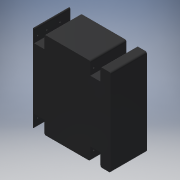
# Autodesk Inventor part: Part2
Saved by Autodesk Inventor 2016 (Build 200138000, 138)
## iProperties
Created: 2015-06-07
Part Number: Part2
Material: ABS Plastic
Document SubType Name: Sheet Metal
Designer: Jufo
Density: 1 g/cm^3
Sheet Metal Rule: Default
Appearance: Smooth - White
Author: Jufo
Autodesk Inventor part; units mm, degrees
ref_plane "YZ Plane" through (0, 0, 0) normal (1, 0, 0) x (0, 1, 0)
ref_plane "XZ Plane" through (0, 0, 0) normal (0, 1, 0) x (-1, 0, 0)
ref_plane "XY Plane" through (0, 0, 0) normal (0, 0, 1) x (1, 0, 0)
sketch "Sketch1" plane through (0, 0, 0) normal (0, 1, 0) x (-1, 0, 0)
  line L0 (65.7605, 110.8282) -> (65.7605, 85.8282)
  line L1 (65.7605, 85.8282) -> (45.7605, 85.8282)
  line L2 (45.7605, 85.8282) -> (45.7605, 110.8282)
  line L3 (45.7605, 110.8282) -> (-44.2395, 110.8282)
  line L4 (-44.2395, 110.8282) -> (-44.2395, 85.8282)
  line L5 (-44.2395, 85.8282) -> (-64.2395, 85.8282)
  line L6 (-64.2395, 85.8282) -> (-64.2395, 110.8282)
  line L7 (-64.2395, 110.8282) -> (-84.2395, 110.8282)
  line L8 (-84.2395, 110.8282) -> (-84.2395, -59.1718)
  line L9 (-84.2395, -59.1718) -> (-64.2395, -59.1718)
  line L10 (-64.2395, -59.1718) -> (-64.2395, -34.1718)
  line L11 (-64.2395, -34.1718) -> (-44.2395, -34.1718)
  line L12 (-44.2395, -34.1718) -> (-44.2395, -59.1718)
  line L13 (-44.2395, -59.1718) -> (45.7605, -59.1718)
  line L14 (45.7605, -59.1718) -> (45.7605, -34.1718)
  line L15 (45.7605, -34.1718) -> (65.7605, -34.1718)
  line L16 (65.7605, -34.1718) -> (65.7605, -59.1718)
  line L17 (65.7605, 110.8282) -> (67.7605, 110.8282)
  line L18 (67.7605, 110.8282) -> (67.7605, -59.1718)
  line L19 (67.7605, -59.1718) -> (65.7605, -59.1718)
  point P0 (0, 0)
  dimension "d0" = 2
  dimension "d1" = 20
  dimension "d2" = 20
  dimension "d3" = 170
  dimension "d4" = 170
  dimension "d6" = 25
  dimension "d9" = 25
  dimension "d10" = 25
  dimension "d11" = 25
  dimension "d12" = 20
  dimension "d13" = 90
  dimension "d14" = 20
  dimension "d15" = 2
  dimension "d16" = 90
  dimension "d17" = 20
  dimension "d113" = 25
  dimension "d114" = 25
  dimension "d115" = 25
  constraints: 40 end point, 14 parallel, 3 perpendicular, 2 collinear, 1 vertical
  measures "d0" distance of L0.start L17.end
  measures "d1" distance of L14.end L15.end
  measures "d2" distance of L0.end L1.end
  measures "d3" distance of L17.end L18.end
  measures "d4" distance of L7.end L8.end
  measures "d6" distance of L13.end L14.end
  measures "d9" distance of L5.end L6.end
  measures "d10" distance of L9.end L10.end
  measures "d11" distance of L11.end L12.end
  measures "d12" distance of L6.end L7.end
  measures "d13" distance of L2.end L3.end
  measures "d14" distance of L8.end L9.end
  measures "d15" distance of L18.end L16.end
  measures "d16" distance of L12.end L13.end
  measures "d17" distance of L10.end L11.end
  measures "d113" distance of L1.end L2.end
  measures "d114" distance of L3.end L4.end
  measures "d115" distance of L0.start L0.end
extrude "Extrusion1" add sketch "Sketch1" along normal blind 2
sketch "Sketch2" plane through (0, 2, 0) normal (0, 1, 0) x (1, 0, 0)
  line L0 (-65.7605, -110.8282) -> (-65.7605, -85.8282) projected
  line L1 (-65.7605, -85.8282) -> (-45.7605, -85.8282) projected
  line L2 (-45.7605, -85.8282) -> (-45.7605, -110.8282) projected
  line L3 (-45.7605, -110.8282) -> (44.2395, -110.8282) projected
  line L4 (44.2395, -110.8282) -> (44.2395, -85.8282) projected
  line L5 (44.2395, -85.8282) -> (64.2395, -85.8282) projected
  line L6 (64.2395, -85.8282) -> (64.2395, -110.8282) projected
  line L7 (64.2395, -110.8282) -> (84.2395, -110.8282) projected
  line L8 (84.2395, -110.8282) -> (84.2395, 59.1718) projected
  line L9 (84.2395, 59.1718) -> (64.2395, 59.1718) projected
  line L10 (64.2395, 59.1718) -> (64.2395, 34.1718) projected
  line L11 (64.2395, 34.1718) -> (44.2395, 34.1718) projected
  line L12 (44.2395, 34.1718) -> (44.2395, 59.1718) projected
  line L13 (44.2395, 59.1718) -> (-45.7605, 59.1718) projected
  line L14 (-45.7605, 59.1718) -> (-45.7605, 34.1718) projected
  line L15 (-45.7605, 34.1718) -> (-65.7605, 34.1718) projected
  line L16 (-65.7605, 34.1718) -> (-65.7605, 59.1718) projected
  line L17 (-65.7605, 59.1718) -> (-67.7605, 59.1718) projected
  line L18 (-67.7605, 59.1718) -> (-67.7605, -110.8282) projected
  line L19 (-67.7605, -110.8282) -> (-65.7605, -110.8282) projected
  line L20 (-67.7605, -81.8282) -> (-43.7605, -81.8282)
  line L21 (-43.7605, -81.8282) -> (-43.7605, -108.8282)
  line L22 (-43.7605, -108.8282) -> (42.2395, -108.8282)
  line L23 (42.2395, -108.8282) -> (42.2395, -81.8282)
  line L24 (42.2395, -81.8282) -> (66.2395, -81.8282)
  line L25 (66.2395, -81.8282) -> (66.2395, -108.8282)
  line L26 (66.2395, -108.8282) -> (82.2395, -108.8282)
  line L27 (82.2395, -108.8282) -> (82.2395, 57.1718)
  line L28 (82.2395, 57.1718) -> (66.2395, 57.1718)
  line L29 (66.2395, 57.1718) -> (66.2395, 30.1718)
  line L30 (66.2395, 30.1718) -> (42.2395, 30.1718)
  line L31 (42.2395, 30.1718) -> (42.2395, 57.1718)
  line L32 (42.2395, 57.1718) -> (-43.7605, 57.1718)
  line L33 (-43.7605, 57.1718) -> (-43.7605, 30.1718)
  line L34 (-43.7605, 30.1718) -> (-67.7605, 30.1718)
  point P0 (0, 0)
  dimension "d20" = 4
  dimension "d21" = 2
  dimension "d22" = 2
  dimension "d23" = 2
  dimension "d26" = 4
  dimension "d27" = 2
  dimension "d28" = 2
  dimension "d29" = 2
  dimension "d30" = 2
  dimension "d31" = 2
  dimension "d32" = 4
  dimension "d33" = 2
  dimension "d34" = 2
  dimension "d35" = 2
  dimension "d36" = 4
  constraints: 30 end point, 8 parallel, 7 perpendicular, 2 point on line
  measures "d20" distance between parallel lines of L15 L34
  measures "d21" distance between parallel lines of L14 L33
  measures "d22" distance between parallel lines of L13 L32
  measures "d23" distance between parallel lines of L12 L31
  measures "d26" distance between parallel lines of L11 L30
  measures "d27" distance between parallel lines of L10 L29
  measures "d28" distance between parallel lines of L9 L28
  measures "d29" distance between parallel lines of L8 L27
  measures "d30" distance between parallel lines of L7 L26
  measures "d31" distance between parallel lines of L6 L25
  measures "d32" distance between parallel lines of L24 L5
  measures "d33" distance between parallel lines of L23 L4
  measures "d34" distance between parallel lines of L3 L22
  measures "d35" distance between parallel lines of L2 L21
  measures "d36" distance between parallel lines of L1 L20
extrude "Extrusion2" add sketch "Sketch2" along normal blind 69 contours L19 L18 L20 L21 L22 L23 L24 L25 L26 L27 L28 L29 L30 L31 L32 L33 L34 L17 L16 L15 L14 L13 L12 L11 L10 L9 L8 L7 L6 L5 L4 L3 L2 L1 L0
sketch "Sketch4" plane through (0, 2, 0) normal (0, 1, 0) x (1, 0, 0)
  line L0 (-43.7605, 30.1718) -> (-67.7605, 30.1718) projected
  line L1 (-67.7605, 30.1718) -> (-67.7605, -81.8282) projected
  line L2 (-67.7605, -81.8282) -> (-43.7605, -81.8282) projected
  line L3 (-65.7605, 30.1718) -> (-65.7605, -81.8282)
  point P0 (0, 0)
  dimension "d39" = 2
  constraints: 2 end point, 2 point on line, 1 perpendicular
  measures "d39" distance between parallel lines of L3 L1
extrude "Extrusion3" add sketch "Sketch4" along normal blind 10
sketch "Sketch5" plane through (44.2395, 0, -34.1718) normal (1, 0, 0) x (0, 0, -1)
  line L0 (0, 0) -> (0, 71) projected
  line L1 (0, 0) -> (0, 7)
  line L2 (0, 7) -> (10, 7)
  circle A0 centre (10, 7) radius 1.6
  point P0 (-34.1718, 0)
  dimension "d42" = 7
  dimension "d43" = 10
  dimension "d44" = 3.2
  constraints: 4 end point, 1 centre point, 1 coincident, 1 perpendicular, 1 point on line
  measures "d42" distance of L0.start L1.end
  measures "d43" distance of L1.end L2.end
  measures "d44" diameter of A0
extrude "Extrusion4" cut sketch "Sketch5" against normal blind 4
sketch "Sketch6" plane through (64.2395, 0, -59.1718) normal (-1, 0, 0) x (0, 0, 1)
  line L0 (25, 0) -> (25, 71) projected
  line L1 (25, 0) -> (25, 7)
  line L2 (25, 7) -> (15, 7)
  circle A0 centre (15, 7) radius 1.6
  point P0 (59.1718, 0)
  dimension "d47" = 7
  dimension "d48" = 10
  dimension "d49" = 3.2
  constraints: 4 end point, 1 centre point, 1 coincident, 1 perpendicular, 1 point on line
  measures "d47" distance of L0.start L1.end
  measures "d48" distance of L1.end L2.end
  measures "d49" diameter of A0
extrude "Extrusion5" cut sketch "Sketch6" against normal blind 4
sketch "Sketch7" plane through (44.2395, 0, 110.8282) normal (1, 0, 0) x (0, 0, -1)
  line L0 (25, 0) -> (25, 71) projected
  line L1 (0, 0) -> (0, 71) projected
  line L2 (25, 0) -> (25, 7)
  line L3 (25, 7) -> (15, 7)
  circle A0 centre (15, 7) radius 1.6
  point P0 (110.8282, 0)
  dimension "d52" = 7
  dimension "d53" = 10
  dimension "d54" = 3.2
  constraints: 4 end point, 1 centre point, 1 coincident, 1 perpendicular, 1 point on line
  measures "d52" distance of L0.start L2.end
  measures "d53" distance of L2.end L3.end
  measures "d54" diameter of A0
extrude "Extrusion6" cut sketch "Sketch7" against normal blind 4
sketch "Sketch8" plane through (64.2395, 0, 85.8282) normal (-1, 0, 0) x (0, 0, 1)
  line L0 (0, 0) -> (0, 71) projected
  line L1 (0, 0) -> (0, 7)
  line L2 (0, 7) -> (10, 7)
  circle A0 centre (10, 7) radius 1.6
  point P0 (-85.8282, 0)
  dimension "d57" = 7
  dimension "d58" = 10
  dimension "d59" = 3.2
  constraints: 4 end point, 1 centre point, 1 coincident, 1 perpendicular, 1 point on line
  measures "d57" distance of L0.start L1.end
  measures "d58" distance of L1.end L2.end
  measures "d59" diameter of A0
extrude "Extrusion7" cut sketch "Sketch8" against normal blind 4
sketch "Sketch9" plane through (-67.7605, 0, -59.1718) normal (-1, 0, 0) x (0, 0, 1)
  line L0 (0, 0) -> (170, 0) projected
  line L1 (29, 12) -> (29, 71) projected
  line L2 (29, 7) -> (15, 7)
  circle A0 centre (15, 7) radius 1.6
  line L3 (25, 0) -> (25, 71) projected
  point P0 (59.1718, 0)
  dimension "d64" = 3.2
  dimension "d119" = 7
  dimension "d365" = 10
  constraints: 2 end point, 1 centre point, 1 coincident, 1 perpendicular, 1 point on line
  measures "d64" diameter of A0
  measures "d119" distance from line of L0 A0.centre
  measures "d365" distance from line of L2.end L3
extrude "Extrusion8" cut sketch "Sketch9" against normal blind 4
sketch "Sketch10" plane through (-45.7605, 0, -59.1718) normal (-1, 0, 0) x (0, 0, 1)
  line L0 (25, 0) -> (25, 71) projected
  line L1 (25, 0) -> (25, 7)
  line L2 (25, 7) -> (15, 7)
  circle A0 centre (15, 7) radius 1.6
  line L3 (0, 0) -> (25, 0) projected
  point P0 (59.1718, 0)
  dimension "d69" = 3.2
  dimension "d387" = 7
  dimension "d388" = 10
  constraints: 4 end point, 1 centre point, 1 perpendicular, 1 point on line
  measures "d69" diameter of A0
  measures "d387" distance from line of L3 A0.centre
  measures "d388" distance from line of L0 A0.centre
extrude "Extrusion9" cut sketch "Sketch10" against normal blind 4
sketch "Sketch11" plane through (-67.7605, 0, -59.1718) normal (-1, 0, 0) x (0, 0, 1)
  line L0 (0, 0) -> (170, 0) projected
  line L1 (0, 0) -> (0, 71) projected
  line L2 (145, 0) -> (145, 7)
  line L3 (145, 7) -> (155, 7)
  circle A0 centre (155, 7) radius 1.6
  line L4 (145, 0) -> (145, 71) projected
  point P0 (59.1718, 0)
  dimension "d72" = 7
  dimension "d73" = 10
  dimension "d74" = 3.2
  dimension "d364" = 10
  constraints: 4 end point, 1 centre point, 1 coincident, 1 parallel, 1 perpendicular, 1 point on line
  measures "d72" distance of L2.start L2.end
  measures "d73" distance of L2.end L3.end
  measures "d74" diameter of A0
  measures "d364" distance from line of L4 L3.end
extrude "Extrusion10" cut sketch "Sketch11" against normal blind 4
sketch "Sketch12" plane through (-45.7605, 0, 85.8282) normal (-1, 0, 0) x (0, 0, 1)
  line L0 (0, 0) -> (0, 71) projected
  line L1 (0, 0) -> (0, 7)
  line L2 (0, 7) -> (10, 7)
  circle A0 centre (10, 7) radius 1.6
  point P0 (-85.8282, 0)
  dimension "d77" = 7
  dimension "d79" = 3.2
  dimension "d363" = 10
  constraints: 4 end point, 1 centre point, 1 coincident, 1 perpendicular, 1 point on line
  measures "d77" distance of L0.start L1.end
  measures "d79" diameter of A0
  measures "d363" distance from line of L0 A0.centre
extrude "Extrusion11" cut sketch "Sketch12" against normal blind 4
sketch "Sketch13" plane through (-67.7605, 0, -59.1718) normal (-1, 0, 0) x (0, 0, 1)
  line L0 (0, 0) -> (170, 0) projected
  line L1 (29, 12) -> (141, 12) projected
  line L2 (0, 71) -> (29, 71) projected
  line L3 (0, 0) -> (0, 71) projected
  line L4 (85, 12) -> (85, 7)
  circle A0 centre (85, 7) radius 1.5
  line L5 (29, 12) -> (44, 12)
  circle A1 centre (44, 7) radius 1.5
  line L6 (14.5, 71) -> (14.5, 51)
  line L7 (14.5, 0) -> (14.5, 25)
  circle A2 centre (14.5, 25) radius 1.5
  circle A3 centre (14.5, 51) radius 1.5
  circle A4 centre (126, 7) radius 1.5
  circle A5 centre (155.5, 25) radius 1.5
  circle A6 centre (155.5, 51) radius 1.5
  line L8 (170, 0) -> (170, 71) projected
  line L9 (141, 12) -> (141, 71) projected
  point P0 (59.1718, 0)
  dimension "d82" = 5
  dimension "d83" = 3
  dimension "d84" = 15
  dimension "d85" = 3
  dimension "d86" = 20
  dimension "d87" = 25
  dimension "d88" = 3
  dimension "d89" = 3
  dimension "d112" = 25
  dimension "d116" = 29
  dimension "d117" = 14.5
  dimension "d118" = 15
  constraints: 8 end point, 7 centre point, 3 coincident, 3 symmetric about line, 2 midpoint, 2 point on line, 1 collinear, 1 parallel, 1 perpendicular, 3 other
  measures "d82" distance of L4.start L4.end
  measures "d83" diameter of A0
  measures "d84" distance of L1.start L5.end
  measures "d85" diameter of A1
  measures "d86" distance of L6.start L6.end
  measures "d87" distance of L7.start L7.end
  measures "d88" diameter of A2
  measures "d89" diameter of A3
  measures "d112" distance from line of L0 A5.centre
  measures "d116" distance between parallel lines of L8 L9
  measures "d117" distance from line of L8 A5.centre
  measures "d118" distance from line of L9 A4.centre
extrude "Extrusion12" cut sketch "Sketch13" against normal blind 2
sketch "Sketch14" plane through (44.2395, 0, 85.8282) normal (0, 0, 1) x (1, 0, 0)
  line L0 (0, 71) -> (20, 71) projected
  line L1 (0, 0) -> (0, 71) projected
  line L2 (0, 71) -> (0, 64)
  line L3 (0, 64) -> (2.625, 64)
  circle A0 centre (2.625, 64) radius 1.5
  line L4 (10, 71) -> (10, 61.5803)
  circle A1 centre (17.375, 64) radius 1.5
  point P0 (-44.2395, 0)
  dimension "d92" = 7
  dimension "d93" = 2.625
  dimension "d94" = 3
  constraints: 6 end point, 2 centre point, 2 perpendicular, 1 coincident, 1 midpoint, 1 point on line, 1 symmetric about line, 1 other
  measures "d92" distance of L0.start L2.end
  measures "d93" distance of L2.end L3.end
  measures "d94" diameter of A0
extrude "Extrusion13" cut sketch "Sketch14" against normal blind 4
sketch "Sketch15" plane through (-65.7605, 0, 85.8282) normal (0, 0, 1) x (1, 0, 0)
  line L0 (0, 71) -> (20, 71) projected
  line L1 (0, 0) -> (0, 71) projected
  line L2 (0, 71) -> (0, 64)
  line L3 (0, 64) -> (2.625, 64)
  circle A0 centre (2.625, 64) radius 1.5
  line L4 (10, 71) -> (10, 64)
  circle A1 centre (17.375, 64) radius 1.5
  point P0 (65.7605, 0)
  dimension "d97" = 7
  dimension "d98" = 2.625
  dimension "d99" = 3
  constraints: 6 end point, 2 centre point, 2 perpendicular, 1 coincident, 1 midpoint, 1 point on line, 1 symmetric about line, 1 other
  measures "d97" distance of L0.start L2.end
  measures "d98" distance of L2.end L3.end
  measures "d99" diameter of A0
extrude "Extrusion14" cut sketch "Sketch15" against normal blind 4
sketch "Sketch16" plane through (-45.7605, 0, -34.1718) normal (0, 0, -1) x (-1, 0, 0)
  line L0 (0, 71) -> (20, 71) projected
  line L1 (0, 0) -> (0, 71) projected
  line L2 (0, 71) -> (0, 64)
  line L3 (0, 64) -> (2.625, 64)
  circle A0 centre (2.625, 64) radius 1.5
  line L4 (10, 71) -> (10, 64.7558)
  circle A1 centre (17.375, 64) radius 1.5
  point P0 (-45.7605, 0)
  dimension "d102" = 7
  dimension "d103" = 2.625
  dimension "d104" = 3
  constraints: 6 end point, 2 centre point, 2 perpendicular, 1 coincident, 1 midpoint, 1 point on line, 1 symmetric about line, 1 other
  measures "d102" distance of L0.start L2.end
  measures "d103" distance of L2.end L3.end
  measures "d104" diameter of A0
extrude "Extrusion15" cut sketch "Sketch16" against normal blind 4
sketch "Sketch17" plane through (64.2395, 0, -34.1718) normal (0, 0, -1) x (-1, 0, 0)
  line L0 (0, 71) -> (20, 71) projected
  line L1 (0, 0) -> (0, 71) projected
  line L2 (0, 71) -> (0, 64)
  line L3 (0, 64) -> (2.625, 64)
  circle A0 centre (2.625, 64) radius 1.5
  line L4 (10, 71) -> (10, 61.2469)
  circle A1 centre (17.375, 64) radius 1.5
  point P0 (64.2395, 0)
  dimension "d107" = 7
  dimension "d108" = 2.625
  dimension "d109" = 3
  constraints: 6 end point, 2 centre point, 2 perpendicular, 1 coincident, 1 midpoint, 1 point on line, 1 symmetric about line, 1 other
  measures "d107" distance of L0.start L2.end
  measures "d108" distance of L2.end L3.end
  measures "d109" diameter of A0
extrude "Extrusion16" cut sketch "Sketch17" against normal blind 4
sketch "Sketch18" plane through (0, 2, 0) normal (0, 1, 0) x (1, 0, 0)
  line L0 (-43.7605, -108.8282) -> (42.2395, -108.8282) projected
  line L1 (66.2395, -108.8282) -> (82.2395, -108.8282) projected
  line L2 (82.2395, -108.8282) -> (82.2395, 57.1718) projected
  line L3 (82.2395, 57.1718) -> (66.2395, 57.1718) projected
  line L4 (42.2395, 57.1718) -> (-43.7605, 57.1718) projected
  line L5 (82.2395, 57.1718) -> (76.2395, 57.1718)
  line L6 (76.2395, 57.1718) -> (76.2395, 51.1718)
  line L7 (76.2395, 51.1718) -> (82.2395, 51.1718)
  line L8 (76.2395, -108.8282) -> (76.2395, -102.8282)
  line L9 (76.2395, -102.8282) -> (82.2395, -102.8282)
  line L10 (-0.7605, -108.8282) -> (-3.7605, -108.8282)
  line L11 (-3.7605, -108.8282) -> (-3.7605, -102.8282)
  line L12 (-3.7605, -102.8282) -> (2.2395, -102.8282)
  line L13 (2.2395, -102.8282) -> (2.2395, -108.8282)
  line L14 (-3.7605, 57.1718) -> (-3.7605, 51.1718)
  line L15 (-3.7605, 51.1718) -> (2.2395, 51.1718)
  line L16 (2.2395, 51.1718) -> (2.2395, 57.1718)
  point P0 (0, 0)
  dimension "d120" = 6
  dimension "d121" = 6
  dimension "d122" = 6
  dimension "d123" = 3
  dimension "d124" = 6
  dimension "d125" = 6
  dimension "d126" = 6
  dimension "d127" = 6
  dimension "d135" = 6
  constraints: 24 end point, 8 point on line, 6 perpendicular, 4 parallel, 1 midpoint
  measures "d120" distance of L2.end L5.end
  measures "d121" distance of L5.end L6.end
  measures "d122" distance of L8.start L8.end
  measures "d123" distance of L10.start L10.end
  measures "d124" distance of L10.end L11.end
  measures "d125" distance of L11.end L12.end
  measures "d126" distance of L14.start L14.end
  measures "d127" distance of L14.end L15.end
  measures "d135" distance of L8.end L9.end
extrude "Extrusion17" add sketch "Sketch18" along normal blind 67
sketch "Sketch19" plane through (0, 71, 0) normal (0, 1, 0) x (1, 0, 0)
  circle A0 centre (-0.7605, 54.1718) radius 1.5
  circle A1 centre (-0.7605, -105.8282) radius 1.5
  circle A2 centre (79.2395, -105.8282) radius 1.5
  circle A3 centre (79.2395, 54.1718) radius 1.5
  line L0 (66.2395, 57.1718) -> (76.2395, 57.1718) projected
  line L1 (82.2395, 51.1718) -> (82.2395, -102.8282) projected
  line L2 (76.2395, -108.8282) -> (66.2395, -108.8282) projected
  line L3 (-43.7605, 57.1718) -> (42.2395, 57.1718) projected
  line L4 (42.2395, -108.8282) -> (-43.7605, -108.8282) projected
  point P0 (0, 0)
  point P1 (82.2395, 57.1718)
  point P2 (82.2395, -108.8282)
  dimension "d130" = 3
  dimension "d131" = 3
  dimension "d132" = 3
  dimension "d136" = 3
  dimension "d137" = 3
  dimension "d138" = 3
  dimension "d139" = 3
  dimension "d202" = 3
  dimension "d203" = 3
  constraints: 4 centre point
  measures "d130" diameter of A0
  measures "d131" diameter of A2
  measures "d132" diameter of A3
  measures "d136" distance from line of L1 A3.centre
  measures "d137" distance from line of L0 A3.centre
  measures "d138" distance from line of L1 A2.centre
  measures "d139" distance from line of L2 A2.centre
  measures "d202" distance from line of L4 A1.centre
  measures "d203" distance from line of L3 A0.centre
extrude "Extrusion18" cut sketch "Sketch19" against normal blind 67
sketch "Sketch33" plane through (42.2395, 2, -30.1718) normal (0, 0, 1) x (1, 0, 0)
  line L0 (24, 0) -> (0, 0) projected
  line L1 (0, 0) -> (0, 69) projected
  line L2 (12, 0) -> (12, 11)
  line L3 (12, 11) -> (9.5, 11)
  line L4 (9.5, 11) -> (9.5, 16)
  line L5 (9.5, 16) -> (14.5, 16)
  line L6 (14.5, 16) -> (14.5, 11)
  line L7 (14.5, 11) -> (12, 11)
  point P0 (-42.2395, -2)
  dimension "d299" = 11
  dimension "d300" = 2.5
  dimension "d301" = 5
  dimension "d302" = 5
  constraints: 12 end point, 3 parallel, 3 perpendicular, 1 midpoint
  measures "d299" distance of L2.start L2.end
  measures "d300" distance of L2.end L3.end
  measures "d301" distance of L3.end L4.end
  measures "d302" distance of L4.end L5.end
extrude "Extrusion32" cut sketch "Sketch33" against normal blind 4
sketch "Sketch34" plane through (66.2395, 2, 81.8282) normal (0, 0, -1) x (-1, 0, 0)
  line L0 (27.5, 0) -> (-0.5, 0)
  line L1 (-0.5, 0) -> (-0.5, 69)
  line L2 (13.5, 0) -> (13.5, 11)
  line L3 (13.5, 11) -> (11, 11)
  line L4 (11, 11) -> (11, 16)
  line L5 (11, 16) -> (16, 16)
  line L6 (16, 16) -> (16, 11)
  line L7 (16, 11) -> (13.5, 11)
  point P0 (66.2395, -2)
  point P1 (-40.2395, -2)
  dimension "d305" = 11
  dimension "d306" = 2.5
  dimension "d307" = 5
  dimension "d308" = 5
  constraints: 16 end point, 3 parallel, 3 perpendicular, 1 midpoint
  measures "d305" distance of L2.start L2.end
  measures "d306" distance of L2.end L3.end
  measures "d307" distance of L3.end L4.end
  measures "d308" distance of L4.end L5.end
extrude "Extrusion33" cut sketch "Sketch34" against normal blind 4
sketch "Sketch35" plane through (-43.7605, 71, 81.8282) normal (0, 0, -1) x (-1, 0, 0)
  line L0 (24, -59) -> (24, 0) projected
  line L1 (0, -69) -> (0, 0) projected
  line L2 (22, -69) -> (0, -69) projected
  line L3 (24, -39.5737) -> (11, -39.5737)
  line L4 (13, -69) -> (13, -58)
  line L5 (13, -58) -> (10.5, -58)
  line L6 (10.5, -58) -> (10.5, -53)
  line L7 (10.5, -53) -> (15.5, -53)
  line L8 (15.5, -53) -> (15.5, -58)
  line L9 (15.5, -58) -> (13, -58)
  point P0 (-43.7605, -71)
  dimension "d311" = 11
  dimension "d312" = 2.5
  dimension "d313" = 5
  dimension "d314" = 5
  constraints: 14 end point, 3 parallel, 3 perpendicular, 2 point on line, 1 collinear
  measures "d311" distance of L4.start L4.end
  measures "d312" distance of L4.end L5.end
  measures "d313" distance of L5.end L6.end
  measures "d314" distance of L6.end L7.end
extrude "Extrusion34" cut sketch "Sketch35" against normal blind 4
sketch "Sketch36" plane through (-67.7605, 71, -30.1718) normal (0, 0, 1) x (1, 0, 0)
  line L0 (26, -59) -> (26, 0)
  line L1 (0, -69) -> (0, 0)
  line L2 (24, -69) -> (0, -69)
  line L3 (26, -39.5737) -> (13, -39.5737)
  line L4 (13, -69) -> (13, -58)
  line L5 (13, -58) -> (10.5, -58)
  line L6 (10.5, -58) -> (10.5, -53)
  line L7 (10.5, -53) -> (15.5, -53)
  line L8 (15.5, -53) -> (15.5, -58)
  line L9 (15.5, -58) -> (13, -58)
  point P0 (67.7605, -71)
  point P1 (-41.7605, -71)
  dimension "d317" = 11
  dimension "d318" = 2.5
  dimension "d319" = 5
  dimension "d320" = 5
  constraints: 20 end point, 3 parallel, 3 perpendicular, 2 point on line, 1 collinear
  measures "d317" distance of L4.start L4.end
  measures "d318" distance of L4.end L5.end
  measures "d319" distance of L5.end L6.end
  measures "d320" distance of L6.end L7.end
extrude "Extrusion35" cut sketch "Sketch36" against normal blind 4
sketch "Sketch55" plane through (0, 2, 0) normal (0, 1, 0) x (1, 0, 0)
  circle A0 centre (38.2395, 53.1718) radius 1.5
  circle A1 centre (-39.7605, 53.1718) radius 1.5
  circle A2 centre (38.2395, -104.8282) radius 1.5
  circle A3 centre (-39.7605, -104.8282) radius 1.5
  line L0 (42.2395, -108.8282) -> (-43.7605, -108.8282) projected
  line L1 (-43.7605, -81.8282) -> (-43.7605, -108.8282) projected
  line L2 (-43.7605, 30.1718) -> (-43.7605, 57.1718) projected
  line L3 (42.2395, -108.8282) -> (34.2395, -108.8282)
  line L4 (34.2395, -108.8282) -> (34.2395, -100.8282)
  line L5 (34.2395, -100.8282) -> (42.2395, -100.8282)
  line L6 (42.2395, -100.8282) -> (42.2395, -108.8282)
  line L7 (-43.7605, -108.8282) -> (-35.7605, -108.8282)
  line L8 (-35.7605, -108.8282) -> (-35.7605, -100.8282)
  line L9 (-35.7605, -100.8282) -> (-43.7605, -100.8282)
  line L10 (-43.7605, -100.8282) -> (-43.7605, -108.8282)
  line L11 (-43.7605, 57.1718) -> (-35.7605, 57.1718)
  line L12 (-35.7605, 57.1718) -> (-35.7605, 49.1718)
  line L13 (-35.7605, 49.1718) -> (-43.7605, 49.1718)
  line L14 (-43.7605, 49.1718) -> (-43.7605, 57.1718)
  line L15 (42.2395, 57.1718) -> (34.2395, 57.1718)
  line L16 (34.2395, 57.1718) -> (34.2395, 49.1718)
  line L17 (34.2395, 49.1718) -> (42.2395, 49.1718)
  line L18 (42.2395, 49.1718) -> (42.2395, 57.1718)
  point P0 (0, 0)
  point P1 (0, 0)
  dimension "d412" = 3
  dimension "d415" = 158
  dimension "d416" = 78
  dimension "d417" = 158
  dimension "d418" = 78
  dimension "d419" = 4
  dimension "d421" = 4
  dimension "d422" = 4
  dimension "d423" = 4
  dimension "d424" = 8
  dimension "d425" = 8
  dimension "d426" = 8
  dimension "d427" = 8
  dimension "d428" = 8
  dimension "d429" = 8
  dimension "d430" = 8
  dimension "d431" = 8
  constraints: 32 end point, 8 parallel, 4 centre point, 4 horizontal, 4 perpendicular, 1 point on line
  measures "d412" diameter of A0
  measures "d415" distance of A1.centre A3.centre
  measures "d416" distance of A0.centre A1.centre
  measures "d417" distance of A2.centre A0.centre
  measures "d418" distance of A2.centre A3.centre
  measures "d419" distance from line of L0 A2.centre
  measures "d421" distance from line of L1 A3.centre
  measures "d422" distance from line of L2 A1.centre
  measures "d423" distance from line of L0 A3.centre
  measures "d424" distance of L4.end L5.end
  measures "d425" distance of L3.end L4.end
  measures "d426" distance of L9.end L8.end
  measures "d427" distance of L8.end L7.end
  measures "d428" distance of L12.end L13.end
  measures "d429" distance of L11.end L12.end
  measures "d430" distance of L17.end L16.end
  measures "d431" distance of L16.end L15.end
extrude "Extrusion53" add sketch "Sketch55" along normal blind 24
fillet "Fillet1" radius 3 10 edges at (84.2395, 35.5, 110.8282) (84.2395, 35.5, -59.1718) (64.2395, 35.5, 110.8282) (44.2395, 35.5, 110.8282) (-45.7605, 35.5, 110.8282) (-65.7605, 35.5, 110.8282) (44.2395, 35.5, -59.1718) (64.2395, 35.5, -59.1718) (-45.7605, 35.5, -59.1718) (-65.7605, 35.5, -59.1718)
sketch "Sketch56" plane through (42.2395, 2, 81.8282) normal (-1, 0, 0) x (0, 0, 1)
  line L0 (19, 0) -> (0, 0) projected
  circle A0 centre (14, 5) radius 1.6 projected
  line L1 (19, 0) -> (19, 10)
  line L2 (19, 0) -> (19, 24) projected
  line L3 (-131, 0) -> (-131, 10)
  line L4 (-131, 24) -> (-131, 0) projected
  line L5 (-121, 0) -> (-131, 0)
  line L6 (9, 0) -> (19, 0)
  line L7 (26, -2) -> (4, -2) projected
  circle A1 centre (-126, 5) radius 1.6 projected
  circle A2 centre (-126, 5) radius 1.5318
  line L8 (-131, 10) -> (-112, 10)
  line L9 (-112, 10) -> (-112, 0)
  line L10 (-131, 0) -> (-131, 24) projected
  line L11 (-112, 0) -> (-131, 0)
  line L12 (19, 10) -> (0, 10)
  line L13 (0, 0) -> (0, 69) projected
  line L14 (0, 10) -> (0, 0)
  line L15 (0, 0) -> (19, 0)
  point P0 (-81.8282, -2)
  dimension "d435" = 5
  dimension "d436" = 10
  dimension "d437" = 5
  dimension "d439" = 10
  constraints: 20 end point, 4 point on line, 2 collinear, 2 horizontal, 2 perpendicular, 1 centre point, 1 coincident, 1 parallel
  measures "d435" distance from line of L0 A0.centre
  measures "d436" distance of L0.start L1.end
  measures "d437" distance from line of L1 A0.centre
  measures "d439" distance of L3.start L3.end
extrude "Extrusion54" add sketch "Sketch56" along normal blind 2 contours L0 L13 L12 L1 | L3 L8 L9 L11 L5
sketch "Sketch57" plane through (-43.7605, 2, 81.8282) normal (1, 0, 0) x (0, 0, -1)
  line L0 (-19, 0) -> (-19, 10)
  line L1 (-19, 0) -> (-19, 24) projected
  line L2 (-19, 10) -> (0, 10)
  line L3 (0, 0) -> (0, 69) projected
  circle A0 centre (-14, 5) radius 1.6 projected
  circle A1 centre (-14, 5) radius 1.7106
  line L4 (0, 0) -> (-19, 0) projected
  line L5 (-19, 0) -> (0, 0)
  line L6 (0, 0) -> (0, 10)
  line L7 (0, 10) -> (0, 0)
  line L8 (131, 0) -> (112, 0) projected
  line L9 (131, 0) -> (131, 10)
  line L10 (131, 0) -> (131, 24) projected
  line L11 (131, 10) -> (112, 10)
  line L12 (112, 0) -> (112, 69) projected
  circle A2 centre (126, 5) radius 1.6 projected
  circle A3 centre (126, 5) radius 1.5
  point P0 (81.8282, -2)
  dimension "d443" = 10
  dimension "d444" = 19
  constraints: 14 end point, 4 point on line, 2 centre point, 2 coincident, 2 collinear, 2 perpendicular, 1 horizontal
  measures "d443" distance of L0.start L0.end
  measures "d444" distance of L0.end L2.end
extrude "Extrusion55" add sketch "Sketch57" along normal blind 2 contours L0 L2 L3 L4 | L8 L12 L11 L9
sketch "Sketch58" plane through (66.2395, 2, 108.8282) normal (1, 0, 0) x (0, 0, -1)
  line L0 (27, 0) -> (0, 0) projected
  line L1 (27, 0) -> (27, 10)
  line L2 (27, 0) -> (27, 69) projected
  line L3 (0, 0) -> (0, 10)
  line L4 (0, 0) -> (0, 69) projected
  line L5 (0, 10) -> (27, 10)
  circle A0 centre (13, 5) radius 1.6 projected
  circle A1 centre (13, 5) radius 1.5
  line L6 (0, -1.4874) -> (27, -0.5674)
  line L7 (166, 0) -> (139, 0) projected
  line L8 (139, 0) -> (139, 10)
  line L9 (139, 0) -> (139, 69) projected
  line L10 (139, 10) -> (166, 10)
  line L11 (166, 0) -> (166, 69) projected
  line L12 (166, 10) -> (166, 0)
  line L13 (166, 0) -> (139, 0)
  circle A2 centre (153, 5) radius 1.6 projected
  circle A3 centre (153, 5) radius 1.5
  point P0 (108.8282, -2)
  dimension "d447" = 10
  dimension "d449" = 10
  constraints: 16 end point, 4 point on line, 2 centre point, 2 coincident, 2 collinear, 2 perpendicular
  measures "d447" distance of L0.start L1.end
  measures "d449" distance of L7.end L8.end
extrude "Extrusion56" add sketch "Sketch58" along normal blind 2 contours L0 L3 L5 L1 | L7 L8 L10 L11
equation "\"d20\" = d36"
equation "\"d28\" = d29"
equation "\"d29\" = d34"
equation "\"d30\" = d22"
equation "\"d34\" = d30"
body "Solid1"
